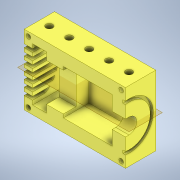
# Autodesk Inventor part: caseLowerPortionV03
Saved by Autodesk Inventor 2022.2 (Build 262287000, 287)
## iProperties
Created: 2021-08-20
Part Number: caseLowerPortionV03
Material: PC/ABS Plastic
Document SubType Name: Modeling
Designer: robst
Density: 0.357273 g/cm^3
Appearance: Smooth - Yellow
Author: robst
Autodesk Inventor part; units mm, degrees
ref_plane "YZ Plane" through (0, 0, 0) normal (1, 0, 0) x (0, 1, 0)
ref_plane "XY Plane" through (0, 0, 0) normal (0, 0, 1) x (1, 0, 0)
sketch "Sketch1" plane through (0, 0, 0) normal (0, 0, 1) x (1, 0, 0)
  line L0 (-60.1, -41.5) -> (60.1, -41.5)
  line L1 (60.1, -41.5) -> (60.1, 41.5)
  line L2 (60.1, 41.5) -> (-60.1, 41.5)
  line L3 (-60.1, 41.5) -> (-60.1, -41.5)
  line L4 (-60.1, -41.5) -> (60.1, 41.5) construction
  line L5 (60.1, -41.5) -> (-60.1, 41.5) construction
  point P0 (0, 0)
  dimension "d0" = 120.2
  dimension "d1" = 83
  constraints: 12 end point, 2 midpoint, 2 parallel, 1 horizontal, 1 perpendicular
  measures "d0" distance of L0.start L0.end
  measures "d1" distance of L1.end L0.end
extrude "MainInnerBodyExtrusion" add sketch "Sketch1" against normal blind 36
sketch "Sketch3" plane through (0, 0, 0) normal (0, 0, 1) x (1, 0, 0)
  line L0 (-13.6, -26.5) -> (44.4, -26.5)
  line L1 (44.4, -26.5) -> (44.4, 26.5)
  line L2 (44.4, 26.5) -> (-13.6, 26.5)
  line L3 (-13.6, 26.5) -> (-13.6, -26.5)
  line L4 (-13.6, -26.5) -> (44.4, 26.5) construction
  line L5 (44.4, -26.5) -> (-13.6, 26.5) construction
  line L6 (60.1, -41.5) -> (60.1, 41.5) projected
  line L7 (0, 0) -> (60.1, 0) construction
  line L8 (-60.1, -41.5) -> (-60.1, 41.5) construction
  line L9 (-60.1, 41.5) -> (-60.1, -41.5) projected
  point P0 (15.4, 0)
  point P1 (15.4, 0)
  dimension "d5" = 15.7
  dimension "d6" = 53
  dimension "d7" = 58
  constraints: 14 end point, 4 midpoint, 2 parallel, 1 horizontal, 1 perpendicular, 1 point on line
  measures "d5" distance between parallel lines of L1 L6
  measures "d6" distance of L0.end L1.end
  measures "d7" distance of L1.end L2.end
extrude "HoleForCameraCase" cut sketch "Sketch3" against normal blind 30.375
sketch "Sketch4" plane through (0, 0, 0) normal (0, 0, 1) x (1, 0, 0)
  line L0 (0, 0) -> (-60.1, 0) construction
  line L1 (-60.1, -41.5) -> (-60.1, 41.5) construction
  line L2 (-50.1, -31.5) -> (-33.6, -31.5)
  line L3 (-33.6, -31.5) -> (-33.6, 31.5)
  line L4 (-33.6, 31.5) -> (-50.1, 31.5)
  line L5 (-50.1, 31.5) -> (-50.1, -31.5)
  line L6 (-50.1, -31.5) -> (-33.6, 31.5) construction
  line L7 (-33.6, -31.5) -> (-50.1, 31.5) construction
  point P0 (-41.85, 0)
  dimension "d13" = 16.5
  dimension "d14" = 63
  dimension "d15" = 10
  constraints: 14 end point, 3 midpoint, 2 parallel, 1 perpendicular, 1 point on line
  measures "d13" distance of L2.start L2.end
  measures "d14" distance of L3.end L2.end
  measures "d15" distance between parallel lines of L1 L5
extrude "HoleForFan" cut sketch "Sketch4" against normal blind 31.5
sketch "Sketch15" plane through (-60.1, -41.5, 0) normal (-1, 0, 0) x (0, 0, 1)
  line L0 (0, 83) -> (0, 0) projected
  line L1 (0, 83) -> (-36, 83) projected
  line L2 (-36, 0) -> (-36, 83) projected
  line L3 (0, 0) -> (-36, 0) projected
  line L4 (0, 0) -> (0, 83) projected
  line L5 (0, 68) -> (0, 15) projected
  line L6 (0, 41.5) -> (-30, 41.5) construction
  line L7 (0, 43.5) -> (-29.9333, 43.5)
  line L8 (0, 51.5) -> (-28.2843, 51.5)
  line L9 (0, 47.5) -> (-29.3939, 47.5)
  line L10 (0, 43.5) -> (0, 41.5)
  line L11 (0, 55.5) -> (-26.533, 55.5)
  line L12 (0, 59.5) -> (-24, 59.5)
  line L13 (-20.4939, 64) -> (0, 64)
  line L14 (-14.9666, 68) -> (0, 68)
  line L15 (0, 51.5) -> (0, 47.5)
  line L16 (0, 68) -> (0, 64)
  line L17 (0, 59.5) -> (0, 55.5)
  line L18 (0, 39.5) -> (-29.9333, 39.5)
  line L19 (0, 31.5) -> (-28.2843, 31.5)
  line L20 (0, 35.5) -> (-29.3939, 35.5)
  line L21 (0, 39.5) -> (0, 41.5)
  line L22 (0, 27.5) -> (-26.533, 27.5)
  line L23 (0, 23.5) -> (-24, 23.5)
  line L24 (-20.4939, 19) -> (0, 19)
  line L25 (-14.9666, 15) -> (0, 15)
  line L26 (0, 31.5) -> (0, 35.5)
  line L27 (0, 23.5) -> (0, 27.5)
  line L28 (0, 15) -> (0, 19)
  line L29 (0, 39.5) -> (0, 43.5)
  line L30 (0, 47.5) -> (0, 51.5)
  line L31 (0, 55.5) -> (0, 59.5)
  line L32 (0, 64) -> (0, 83)
  arc A0 (-28.2843, 51.5) -> (-29.3939, 47.5) centre (0, 41.5) ccw
  arc A1 (-14.9666, 68) -> (-20.4939, 64) centre (0, 41.5) ccw
  arc A2 (-24, 59.5) -> (-26.533, 55.5) centre (0, 41.5) ccw
  arc A3 (-29.9333, 43.5) -> (-29.9333, 39.5) centre (0, 41.5) ccw
  arc A4 (-29.3939, 35.5) -> (-28.2843, 31.5) centre (0, 41.5) ccw
  arc A5 (-26.533, 27.5) -> (-24, 23.5) centre (0, 41.5) ccw
  arc A6 (-20.4939, 19) -> (-14.9666, 15) centre (0, 41.5) ccw
  point P0 (0, 41.5)
  point P1 (0, 82)
  point P2 (0, 67.0167)
  point P3 (0, 4.25)
  point P4 (-10.247, 64)
  point P5 (0, 15)
  point P6 (0, 19)
  point P7 (0, 23.5)
  point P8 (0, 27.5)
  point P9 (0, 31.5)
  point P10 (0, 35.5)
  point P11 (0, 39.5)
  point P12 (0, 47.5)
  point P13 (0, 51.5)
  point P14 (0, 55.5)
  point P15 (0, 59.5)
  point P16 (0, 64)
  dimension "d69" = 2
  dimension "d71" = 4
  dimension "d72" = 4
  dimension "d73" = 4
  dimension "d75" = 4
  dimension "d142" = 30
  constraints: 54 end point, 15 point on circle, 15 symmetric about line, 7 centre point, 3 parallel, 3 perpendicular, 2 horizontal, 1 coincident, 1 midpoint, 1 other
  measures "d69" distance between parallel lines of L7 L6
  measures "d71" distance between parallel lines of L8 L9
  measures "d72" distance between parallel lines of L11 L8
  measures "d73" distance between parallel lines of L12 L11
  measures "d75" distance between parallel lines of L13 L14
  measures "d142" radius of A2
extrude "SlotsForRearFan" cut sketch "Sketch15" against normal up to surface (10 mm away) contours L0 L13 A1 L14 | L0 L11 A2 L12 | L25 A6 L24 L0 | L0 L9 A0 L8 | L23 A5 L22 L0 | L0 L18 A3 L7 | L19 A4 L20 L0
sketch "Sketch16" plane through (0, 0, -30.375) normal (0, 0, 1) x (1, 0, 0)
  line L0 (44.4, 26.5) -> (44.4, -26.5) projected
  line L1 (28.9, 10.765) -> (28.9, -11.235) construction
  line L2 (27.4, 10.765) -> (27.4, -11.235)
  line L3 (24.4, -11.235) -> (24.4, 10.765)
  line L4 (21.4, 8.7746) -> (21.4, -9.2446)
  line L5 (18.4, 3.5785) -> (18.4, -4.0485)
  line L6 (30.4, 10.765) -> (30.4, -11.235)
  line L7 (33.4, -11.235) -> (33.4, 10.765)
  line L8 (36.4, 8.7746) -> (36.4, -9.2446)
  line L9 (39.4, 3.5785) -> (39.4, -4.0485)
  line L10 (22.5491, 10.765) -> (24.4, 10.765)
  line L11 (24.4, -11.235) -> (22.5491, -11.235)
  line L12 (22.5491, -11.235) -> (21.4, -9.2446)
  line L13 (18.4, -4.0485) -> (16.1983, -0.235)
  line L14 (16.1983, -0.235) -> (18.4, 3.5785)
  line L15 (21.4, 8.7746) -> (22.5491, 10.765)
  line L16 (27.4, 10.765) -> (30.4, 10.765)
  line L17 (33.4, 10.765) -> (35.2509, 10.765)
  line L18 (35.2509, -11.235) -> (33.4, -11.235)
  line L19 (30.4, -11.235) -> (27.4, -11.235)
  line L20 (41.6017, -0.235) -> (39.4, -4.0485)
  line L21 (36.4, -9.2446) -> (35.2509, -11.235)
  line L22 (35.2509, 10.765) -> (36.4, 8.7746)
  line L23 (39.4, 3.5785) -> (41.6017, -0.235)
  point P0 (0, 0)
  point P1 (28.9, -0.235)
  point P2 (18.4, -0.235)
  dimension "d78" = 15.5
  dimension "d89" = 1.5
  dimension "d90" = 3
  dimension "d91" = 3
  dimension "d92" = 3
  constraints: 46 end point, 8 symmetric about line, 6 perpendicular, 3 horizontal, 3 midpoint, 2 vertical, 7 other
  measures "d78" distance from line of point (28.9, -0.235) L0
  measures "d89" distance between parallel lines of L2 L1
  measures "d90" distance between parallel lines of L3 L2
  measures "d91" distance between parallel lines of L4 L3
  measures "d92" distance from line of point (18.4, -0.235) L4
extrude "VentForCamera" cut sketch "Sketch16" against normal through all
sketch "Sketch18" plane through (60.1, -41.5, 0) normal (1, 0, 0) x (0, 0, -1)
  line L0 (0, 41.5) -> (29.6767, 41.5) construction
  arc A0 (4.125, 32.25) -> (4.125, 50.75) centre (4.125, 41.5) ccw
  line L1 (0, 0) -> (0, 83) projected
  line L2 (4.125, 50.75) -> (0, 50.75)
  line L3 (4.125, 32.25) -> (0, 32.25)
  line L4 (0, 50.75) -> (0, 32.25)
  point P0 (0, 41.5)
  dimension "d97" = 18.5
  dimension "d137" = 4.125
  constraints: 8 end point, 3 point on line, 2 perpendicular, 2 point on circle, 2 tangent, 1 centre point, 1 collinear, 1 horizontal, 1 midpoint
  measures "d97" diameter of A0
  measures "d137" distance of point (0, 41.5) A0.centre
extrude "HoleForLens" cut sketch "Sketch18" against normal blind 20
sketch "Sketch23" plane through (0, 0, 0) normal (0, 0, 1) x (1, 0, 0)
  line L0 (-55.1, -36.5) -> (55.1, -36.5) construction
  line L1 (55.1, -36.5) -> (55.1, 36.5) construction
  line L2 (55.1, 36.5) -> (-55.1, 36.5) construction
  line L3 (-55.1, 36.5) -> (-55.1, -36.5) construction
  line L4 (-55.1, -36.5) -> (55.1, 36.5) construction
  line L5 (55.1, -36.5) -> (-55.1, 36.5) construction
  line L6 (60.1, -41.5) -> (60.1, -9.25) projected
  line L7 (60.1, 41.5) -> (-60.1, 41.5) projected
  line L8 (-13.6, -26.5) -> (-13.6, 26.5) projected
  line L9 (-33.6, 31.5) -> (-33.6, -31.5) projected
  line L10 (-33.6, 31.5) -> (-33.6, -31.5) projected
  line L11 (-13.6, 26.5) -> (-33.6, 26.5)
  line L12 (-33.6, 26.5) -> (-33.6, -25.5)
  line L13 (-33.6, -25.5) -> (-13.6, -25.5)
  line L14 (-13.6, -25.5) -> (-13.6, 26.5)
  point P0 (0, 0)
  dimension "d106" = 5
  dimension "d108" = 5
  constraints: 20 end point, 4 coincident, 4 parallel, 2 horizontal, 2 midpoint, 2 perpendicular, 1 point on line
  measures "d106" distance between parallel lines of L1 L6
  measures "d108" distance between parallel lines of L2 L7
hole "Hole for 6-32 Insert" at (-55.1, 36.5, 0) at (55.1, 36.5, 0) at (55.1, -36.5, 0) at (-55.1, -36.5, 0) direction (0, 0, -1) diameter 4.7 depth 7.2 tip angle 118 counterbore diameter 5.54 counterbore depth 5.55
hole "Screw hole for 6-32 screw" at (-55.1, -36.5, 0) at (55.1, -36.5, 0) at (55.1, 36.5, 0) at (-55.1, 36.5, 0) direction (0, 0, -1) diameter 3.797 depth 15 tip angle 118 clearance for "Hex Machine Screw" size "#6" standard "Ansi Unified Screw Threads"
sketch "HoleFor50mmLensCover" plane through (60.1, -41.5, -36) normal (1, 0, 0) x (0, 0, -1)
  arc A0 (-31.875, 32.25) -> (-31.875, 50.75) centre (-31.875, 41.5) ccw projected
  circle A1 centre (-31.125, 41.5) radius 28
  circle A2 centre (-31.125, 41.5) radius 24.5
  line L0 (-70.35, 41.5) -> (11.725, 41.5) projected
  point P0 (-36, 41.5)
  dimension "d163" = 56
  dimension "d164" = 49
  dimension "d179" = 0
  constraints: 2 centre point, 1 coincident
  measures "d163" diameter of A1
  measures "d164" diameter of A2
  measures "d179" distance from line of A1.centre L0
extrude "HoleForLensCover" cut sketch "HoleFor50mmLensCover" against normal blind 3 contours L0 A2 A1 | A1 L0 A2
sketch "Sketch32" plane through (0, 0, 0) normal (0, 0, 1) x (1, 0, 0)
  line L0 (-13.6, -26.5) -> (-13.6, 26.5) projected
  line L1 (-33.6, 31.5) -> (-33.6, -31.5) projected
  line L2 (-13.6, 22.5) -> (-33.6, 22.5)
  line L3 (-33.6, 22.5) -> (-33.6, -22.5)
  line L4 (-33.6, -22.5) -> (-13.6, -22.5)
  line L5 (-13.6, -22.5) -> (-13.6, 22.5)
  line L6 (-13.6, 26.5) -> (44.4, 26.5) projected
  line L7 (44.4, -26.5) -> (-13.6, -26.5) projected
  point P0 (0, 0)
  point P1 (-13.6, -22.5)
  dimension "d180" = 4
  dimension "d181" = 4
  constraints: 8 end point, 2 parallel, 2 point on line, 1 horizontal, 1 perpendicular
  measures "d180" distance between parallel lines of L2 L6
  measures "d181" distance between parallel lines of L4 L7
extrude "Extrusion23" cut sketch "Sketch32" against normal blind 15
sketch "Sketch33" plane through (-60.1, -41.5, 0) normal (0, -1, 0) x (1, 0, 0)
  line L0 (0, 0) -> (0, -36) construction
  line L1 (0, -18) -> (120.2, -18) construction
  line L2 (120.2, 0) -> (120.2, -36) construction
  point P0 (60.1, 0)
  point P1 (11.82, -18)
  point P2 (35.46, -18)
  point P3 (59.1, -18)
  point P4 (82.74, -18)
  point P5 (106.38, -18)
  dimension "d184" = 11.82
  dimension "d187" = 23.64
  constraints: 2 end point, 2 midpoint, 1 horizontal, 1 point on line, 4 other
  measures "d184" distance from line of point (11.82, -18) L0
  measures "d187" distance of point (11.82, -18) point (35.46, -18)
hole "Hole7" at (-48.28, -41.5, -18) at (-24.64, -41.5, -18) at (-1, -41.5, -18) at (22.64, -41.5, -18) at (46.28, -41.5, -18) direction (0, 1, 0) diameter 6.756 depth 9 counterbore diameter 8.1509 counterbore depth 7.4168 clearance for "Hex Machine Screw" size "1/4" standard "Ansi Unified Screw Threads"
mirror "Mirror4" about plane through (0, 0, 0) normal (0, 1, 0) of "Hole7"
equation "\"d0\" = caseLength"
equation "\"d2\" = caseDepth"
equation "\"d5\" = lensLength"
equation "\"d6\" = cameraWidth"
equation "\"d7\" = cameraLength"
equation "\"d13\" = fanDepth"
equation "\"d14\" = fanWidth"
equation "\"d15\" = rearWallThickness"
equation "\"caseWidth\" = 83"
equation "\"lensLength\" = 15.7"
equation "\"lensDiameter\" = 17.5"
equation "\"thickenDistance\" = 1.5"
equation "\"bottomOfCaseWallThickness\" = 3"
equation "\"rearWallThickness\" = 10"
equation "\"maxComponentDepth\" = 33"
equation "\"caseDepth\" = maxComponentDepth + bottomOfCaseWallThickness"
equation "\"fanCutoutDepth\" = 0.5 * fanLength + extraCutoutDepth + thickenDistance"
equation "\"caseLength\" = 120.2"
equation "\"frontWallThickness\" = 3"
equation "\"d95\" = lensDiameter"
equation "\"extraCutoutDepth\" = 15.5"
equation "\"halfFanDepth\" = 31.5"
equation "\"cameraCaseDepth\" = 57.75"
equation "\"halfCameraCaseDepth\" = 30.375"
equation "\"halfThirmesterDepth\" = 11.5"
equation "\"halfSensorDepth\" = 11.5"
equation "\"depthForLensSlot\" = 4.125"
equation "\"bottomWallThickness\" = 8"
equation "\"cameraWidth\" = 53"
equation "\"cameraLength\" = 58"
equation "\"fanDepth\" = 16.5"
equation "\"fanWidth\" = 63"
equation "\"fanLength\" = 60"
body "Solid1"
